rod_end_cap (Autodesk Fusion 360 design; units mm, degrees)
part number: 2026-09-03-23-52-10-226
Autodesk Fusion 360 part; units mm, degrees
sketch "End cap profile" plane through (0, 0, 0) normal (0, 1, 0) x (1, 0, 0)
  line L0 (0, 0) -> (21, 0)
  line L1 (21, 0) -> (21, -4)
  line L2 (21, -4) -> (14.7, -4)
  line L3 (14.7, -4) -> (14.7, -26.5)
  line L4 (14.7, -26.5) -> (13.2, -28)
  line L5 (13.2, -28) -> (0, -28)
  line L6 (0, -28) -> (0, 0)
  dimension "d27" = 21
  dimension "d28" = 4
  dimension "d29" = 14.7
  dimension "d30" = 28
  dimension "d31" = 1.5
  dimension "d32" = 1.5
  constraint horizontal L0
  constraint horizontal L2
  constraint horizontal L5
  constraint vertical L1
  constraint vertical L3
  constraint vertical L6
  constraint coincident L0.start L6.end
  measures "d27" horizontal distance of L0.start L0.end
  measures "d28" vertical distance of L0.end L1.end
  measures "d29" horizontal distance of L0.start L2.end
  measures "d30" vertical distance of L0.start L5.end
  measures "d31" horizontal distance of L3.end L4.end
  measures "d32" vertical distance of L3.end L4.end
revolve "End cap revolve" add sketch "End cap profile" angle 360 about axis through (0, 0, 1.75) along (0, 0, 1)
sketch "Crush rib" plane through (0, 0, 0) normal (0, 1, 0) x (1, 0, 0)
  line L0 (13.7, -5) -> (15.2, -5)
  line L1 (15.2, -5) -> (15.2, -24.5)
  line L2 (15.2, -24.5) -> (13.7, -26)
  line L3 (13.7, -26) -> (13.7, -5)
  dimension "d34" = 13.7
  dimension "d35" = 5
  dimension "d36" = 15.2
  dimension "d37" = 26
  dimension "d38" = 24.5
  constraint horizontal L0
  constraint vertical L1
  constraint vertical L3
  measures "d34" horizontal distance of origin L0.start
  measures "d35" vertical distance of origin L0.start
  measures "d36" horizontal distance of origin L0.end
  measures "d37" vertical distance of origin L2.end
  measures "d38" vertical distance of origin L1.end
extrude "Crush rib (1)" add sketch "Crush rib" along normal mid plane 2
pattern_circular "Crush ribs" count 4 over 360 about axis through (0, 0, 1.75) along (0, 0, 1) of "Crush rib (1)"
equation "rodOuterDiameter = 33.4 mm" comment "drives the model; safe to edit live in Fusion"
equation "pipeInnerDiameter = 30.0 mm" comment "drives the model; safe to edit live in Fusion"
equation "endCapFlangeProud = 4.3 mm" comment "drives the model; safe to edit live in Fusion"
equation "endCapFlangeThickness = 4.0 mm" comment "drives the model; safe to edit live in Fusion"
equation "endCapStemLength = 24.0 mm" comment "drives the model; safe to edit live in Fusion"
equation "endCapStemDiameter = pipeInnerDiameter - 0.6 mm" comment "drives the model; safe to edit live in Fusion"
equation "endCapRibDiameter = pipeInnerDiameter + 0.4 mm" comment "drives the model; safe to edit live in Fusion"
equation "endCapTipChamfer = 1.5 mm" comment "drives the model; safe to edit live in Fusion"
equation "endCapRibWidth = 2.0 mm" comment "drives the model; safe to edit live in Fusion"
equation "endCapRibCount = 4" comment "drives the model; safe to edit live in Fusion"
equation "d27 = rodOuterDiameter / 2 + endCapFlangeProud"
equation "d28 = endCapFlangeThickness"
equation "d29 = endCapStemDiameter / 2"
equation "d30 = endCapFlangeThickness + endCapStemLength"
equation "d31 = endCapTipChamfer"
equation "d32 = endCapTipChamfer"
equation "d34 = endCapStemDiameter / 2 - 1 mm"
equation "d35 = endCapFlangeThickness + 1 mm"
equation "d36 = endCapRibDiameter / 2"
equation "d37 = endCapFlangeThickness + endCapStemLength - 2 mm"
equation "d38 = endCapFlangeThickness + endCapStemLength - 3.5 mm"
equation "d39 = endCapRibWidth"
equation "d41 = endCapRibCount"
named bodies: "rod_end_cap"
